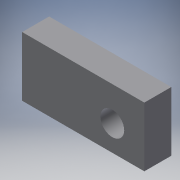
# Autodesk Inventor part: Fixer
Saved by Autodesk Inventor 2019 (Build 230136000, 136)
## iProperties
Created: 2021-11-07
Part Number: Fixer
Material: Generic
Document SubType Name: Modeling
Designer: Mohamed Teleb
Density: 1 g/cm^3
Appearance: Default
Author: Mohamed Teleb
Autodesk Inventor part; units mm, degrees
ref_plane "YZ Plane" through (0, 0, 0) normal (1, 0, 0) x (0, 1, 0)
ref_plane "XZ Plane" through (0, 0, 0) normal (0, 1, 0) x (-1, 0, 0)
ref_plane "XY Plane" through (0, 0, 0) normal (0, 0, 1) x (1, 0, 0)
sketch "Sketch1" plane through (0, 0, 0) normal (0, 0, 1) x (1, 0, 0)
  line L0 (-21.2538, 6.4099) -> (9.5462, 6.4099)
  line L1 (9.5462, 6.4099) -> (9.5462, -8.5901)
  line L2 (9.5462, -8.5901) -> (-21.2538, -8.5901)
  line L3 (-21.2538, -8.5901) -> (-21.2538, 6.4099)
  line L4 (1.0462, -38.9134) -> (26.8462, -38.9134)
  line L5 (-4.9538, -50.9134) -> (0.0462, -50.9134)
  point P0 (0, 0)
  dimension "d0" = 30.8
  dimension "d1" = 15
  dimension "d8" = 25.8
  dimension "d9" = 5
  constraints: 12 end point, 3 horizontal, 2 parallel, 1 perpendicular, 4 other
  measures "d0" distance of L1.end L2.end
  measures "d1" distance of L0.end L1.end
  measures "d8" distance of L4.start L4.end
  measures "d9" distance of L5.start L5.end
extrude "Extrusion1" add sketch "Sketch1" along normal blind 6.8
sketch "Sketch2" plane through (0, 0, 6.8) normal (0, 0, 1) x (1, 0, 0)
  circle A0 centre (1.4656, -2.1794) radius 3 projected
  circle A1 centre (1.4656, -2.1794) radius 3
  point P0 (0, 0)
  constraints: 1 centre point, 1 coincident, 1 concentric
extrude "Extrusion2" cut sketch "Sketch2" against normal blind 14
sketch "Sketch3" plane through (0, 0, 0) normal (0, 0, -1) x (-1, 0, 0)
  line L0 (5.4538, -4.4054) -> (8.8538, -4.4054) projected
  line L1 (5.4538, 2.5946) -> (8.8538, 2.5946) projected
  line L2 (8.8538, 84.2919) -> (8.8538, -65.7081) projected
  line L3 (5.4538, -4.4054) -> (8.8538, -4.4054)
  line L4 (8.8538, -4.4054) -> (8.8538, 2.5946)
  line L5 (8.8538, 2.5946) -> (5.4538, 2.5946)
  line L6 (5.4538, 2.5946) -> (5.4538, -4.4054)
  point P0 (0, 0)
  constraints: 8 end point, 2 parallel, 1 horizontal, 1 perpendicular
extrude "Extrusion3" add sketch "Sketch3" against normal blind 3.4
sketch "Sketch4" plane through (-21.2538, -8.5901, 0) normal (-1, 0, 0) x (0, 0, 1)
  line L0 (3.4, 2.3591) -> (0, 2.3591)
  line L1 (3.4, 9.3591) -> (3.4, 2.3591)
  line L2 (3.4, 2.3591) -> (0, 2.3591)
  line L3 (0, 2.3591) -> (0, 9.3591)
  line L4 (0, 9.3591) -> (3.4, 9.3591)
  line L5 (3.4, 9.3591) -> (3.4, 2.3591)
  point P0 (0, 8.5901)
  constraints: 12 end point, 2 horizontal, 2 parallel, 1 perpendicular, 1 vertical, 3 other
extrude "Extrusion4" add sketch "Sketch4" along normal blind 3.4
equation "\"d0\" = d8 + d9"
body "Solid1"
